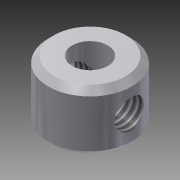
# Autodesk Inventor part: sttopa
Saved by Autodesk Inventor 2015 (Build 190159000, 159)
## iProperties
Created: 2013-10-24
Part Number: sttopa
Material: アルミニウム 2014-T4
Document SubType Name: Modeling
Designer: kenta
Density: 2.8 g/cm^3
Appearance: サテン
Mass: 0.384365 g
Surface Area: 2.3344 cm^2
Volume: 0.137273 cm^3
Author: kenta
Autodesk Inventor part; units mm, degrees
ref_plane "YZ Plane" through (0, 0, 0) normal (1, 0, 0) x (0, 1, 0)
ref_plane "XZ Plane" through (0, 0, 0) normal (0, 1, 0) x (-1, 0, 0)
ref_plane "XY Plane" through (0, 0, 0) normal (0, 0, 1) x (1, 0, 0)
sketch "スケッチ1" plane through (0, 0, 0) normal (0, 0, 1) x (1, 0, 0)
  line L0 (-3.5, 3.5) -> (3.5, 3.5)
  line L1 (3.5, 3.5) -> (3.5, -3.5)
  line L2 (3.5, -3.5) -> (-3.5, -3.5)
  line L3 (-3.5, -3.5) -> (-3.5, 3.5)
  line L4 (-3.5, 3.5) -> (3.5, -3.5) construction
  line L5 (3.5, 3.5) -> (-3.5, -3.5) construction
  point P0 (0, 0)
  dimension "d0" = 7
  dimension "d2" = 7
  constraints: 12 end point, 2 midpoint, 2 parallel, 1 horizontal, 1 perpendicular
  measures "d0" distance between parallel lines of L2 L0
  measures "d2" distance between parallel lines of L3 L1
extrude "押し出し1" add sketch "スケッチ1" along normal blind 5
sketch "スケッチ2" plane through (3.5, -3.5, 0) normal (1, 0, 0) x (0, 0, -1)
  line L0 (-5, 0) -> (-5, 7) projected
  line L1 (0, 0) -> (-5, 0) projected
  point P0 (0, 3.5)
  point P1 (-2.5, 3.5)
  dimension "d5" = 2.5
  dimension "d6" = 3.5
  measures "d5" distance from line of point (-2.5, 3.5) L0
  measures "d6" distance from line of L1 point (-2.5, 3.5)
hole "穴1" at (3.5, 0, 2.5) direction (-1, 0, 0) diameter 2.459 end through all thread size "M3x0.5" class "6H" standard "ANSI Metric M Profile"
sketch "スケッチ3" plane through (0, 0, 5) normal (0, 0, 1) x (1, 0, 0)
  line L0 (3.5, 3.5) -> (-3.5, 3.5) projected
  line L1 (-3.5, 3.5) -> (-3.5, -3.5) projected
  line L2 (-3.5, -3.5) -> (3.5, -3.5) projected
  line L3 (3.5, -3.5) -> (3.5, 3.5) projected
  circle A0 centre (0, 0) radius 3.5
  point P0 (0, 0)
  constraints: 3 tangent, 1 centre point
extrude "押し出し2" cut sketch "スケッチ3" against normal blind 5 contours L3 A0 L0 | A0 L1 L0 | L3 L2 A0 | A0 L2 L1
sketch "スケッチ4" plane through (0, 0, 5) normal (0, 0, 1) x (1, 0, 0)
  circle A0 centre (0, 0) radius 3.5 projected
  circle A1 centre (0, 0) radius 1.5
  dimension "d16" = 3
  constraints: 1 centre point, 1 coincident
  measures "d16" diameter of A1
hole "穴2" at (0, 0, 5) at (0, 0, 5) direction (0, 0, -1) diameter 3 end through all
chamfer "面取り1" distance 0.5 angle 45 2 edges at (-3.5, 0, 0) (-3.5, 0, 5)
